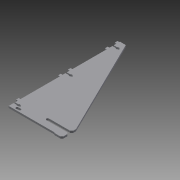
# Autodesk Inventor part: support1
Saved by Autodesk Inventor 2015 SP2 (Build 190223200, 223)
## iProperties
Created: 2016-02-16
Part Number: support1
Material: Generic
Document SubType Name: Modeling
Designer: marc
Density: 1 g/cm^3
Appearance: Default
Author: marc
Autodesk Inventor part; units mm, degrees
ref_plane "YZ Plane" through (0, 0, 0) normal (1, 0, 0) x (0, 1, 0)
ref_plane "XZ Plane" through (0, 0, 0) normal (0, 1, 0) x (-1, 0, 0)
ref_plane "XY Plane" through (0, 0, 0) normal (0, 0, 1) x (1, 0, 0)
sketch "Sketch1" plane through (0, 0, 0) normal (0, 0, 1) x (1, 0, 0)
  line L0 (0, 0) -> (183.9, 0)
  line L1 (183.9, 0) -> (183.9, 47)
  line L2 (183.9, 47) -> (25.4, 370)
  line L3 (25.4, 370) -> (0, 370)
  line L4 (0, 370) -> (0, 0)
  dimension "d0" = 370
  dimension "d1" = 183.9
  dimension "d2" = 25.4
  dimension "d3" = 47
  constraints: 10 end point, 2 perpendicular, 1 horizontal, 1 parallel
  measures "d0" distance between parallel lines of L0 L3
  measures "d1" distance between parallel lines of L1 L4
  measures "d2" distance of L2.end L3.end
  measures "d3" distance of L0.end L1.end
extrude "Extrusion1" add sketch "Sketch1" along normal blind 6
sketch "Sketch2" plane through (0, 0, 6) normal (0, 0, 1) x (1, 0, 0)
  line L0 (0, 370) -> (6, 370)
  line L1 (6, 370) -> (6, 367.743)
  line L2 (6, 367.743) -> (0, 367.743)
  line L3 (0, 367.743) -> (0, 370)
  line L4 (25.4, 370) -> (0, 370) projected
  line L5 (0, 370) -> (0, 0) projected
  line L6 (0, 358.743) -> (6, 358.743)
  line L7 (6, 358.743) -> (6, 335.443)
  line L8 (6, 335.443) -> (0, 335.443)
  line L9 (0, 335.443) -> (0, 358.743)
  line L10 (0, 326.443) -> (6, 326.443)
  line L11 (6, 326.443) -> (6, 212.65)
  line L12 (6, 212.65) -> (0, 212.65)
  line L13 (0, 212.65) -> (0, 326.443)
  line L14 (0, 203.65) -> (6, 203.65)
  line L15 (6, 203.65) -> (6, 180.35)
  line L16 (6, 180.35) -> (0, 180.35)
  line L17 (0, 180.35) -> (0, 203.65)
  line L18 (0, 171.35) -> (6, 171.35)
  line L19 (6, 171.35) -> (6, 41.15)
  line L20 (6, 41.15) -> (0, 41.15)
  line L21 (0, 41.15) -> (0, 171.35)
  line L22 (0, 32.15) -> (6, 32.15)
  line L23 (6, 32.15) -> (6, 0)
  line L24 (6, 0) -> (0, 0)
  line L25 (0, 0) -> (0, 32.15)
  line L26 (0, 0) -> (183.9, 0) projected
  dimension "d6" = 9
  dimension "d7" = 9
  dimension "d8" = 9
  dimension "d9" = 9
  dimension "d12" = 6
  dimension "d14" = 9
  dimension "d53" = 32.15
  dimension "d54" = 171.35
  dimension "d55" = 203.65
  dimension "d56" = 326.443
  dimension "d57" = 358.743
  constraints: 48 end point, 12 parallel, 7 point on line, 6 collinear, 6 horizontal, 6 perpendicular
  measures "d6" distance between parallel lines of L6 L2
  measures "d7" distance between parallel lines of L8 L10
  measures "d8" distance between parallel lines of L22 L20
  measures "d9" distance between parallel lines of L18 L16
  measures "d12" distance between parallel lines of L5 L1
  measures "d14" distance between parallel lines of L12 L14
  measures "d53" distance between parallel lines of L26 L22
  measures "d54" distance between parallel lines of L26 L18
  measures "d55" distance between parallel lines of L26 L14
  measures "d56" distance between parallel lines of L26 L10
  measures "d57" distance between parallel lines of L26 L6
extrude "Extrusion2" cut sketch "Sketch2" against normal through all
sketch "Sketch3" plane through (0, 0, 6) normal (0, 0, 1) x (1, 0, 0)
  line L0 (-10.0727, 347.093) -> (75.5841, 347.093) construction
  line L1 (6, 344.893) -> (27.1, 344.893)
  line L2 (27.1, 344.893) -> (27.1, 349.293)
  line L3 (27.1, 349.293) -> (6, 349.293)
  line L4 (6, 349.293) -> (6, 344.893)
  line L5 (6, 344.893) -> (27.1, 349.293) construction
  line L6 (27.1, 344.893) -> (6, 349.293) construction
  line L7 (6, 358.743) -> (6, 335.443) projected
  line L8 (18, 343.093) -> (23.1, 343.093)
  line L9 (23.1, 343.093) -> (23.1, 351.093)
  line L10 (23.1, 351.093) -> (18, 351.093)
  line L11 (18, 351.093) -> (18, 343.093)
  line L12 (18, 343.093) -> (23.1, 351.093) construction
  line L13 (23.1, 343.093) -> (18, 351.093) construction
  line L14 (25.4, 370) -> (6, 370) projected
  line L15 (-23.1846, 192) -> (187.875, 192) construction
  line L16 (6, 189.8) -> (27.1, 189.8)
  line L17 (27.1, 189.8) -> (27.1, 194.2)
  line L18 (27.1, 194.2) -> (6, 194.2)
  line L19 (6, 194.2) -> (6, 189.8)
  line L20 (6, 189.8) -> (27.1, 194.2) construction
  line L21 (27.1, 189.8) -> (6, 194.2) construction
  line L22 (23.1, 188) -> (18, 188)
  line L23 (18, 188) -> (18, 196)
  line L24 (18, 196) -> (23.1, 196)
  line L25 (23.1, 196) -> (23.1, 188)
  line L26 (23.1, 188) -> (18, 196) construction
  line L27 (18, 188) -> (23.1, 196) construction
  line L28 (6, 203.65) -> (6, 180.35) projected
  line L29 (20.55, 484.1375) -> (20.55, -100.4436) construction
  line L30 (-93.0618, 20.51) -> (253.6101, 20.51) construction
  line L31 (6, 18.31) -> (27.1, 18.31)
  line L32 (27.1, 18.31) -> (27.1, 22.71)
  line L33 (27.1, 22.71) -> (6, 22.71)
  line L34 (6, 22.71) -> (6, 18.31)
  line L35 (6, 18.31) -> (27.1, 22.71) construction
  line L36 (27.1, 18.31) -> (6, 22.71) construction
  line L37 (23.1, 16.51) -> (18, 16.51)
  line L38 (18, 16.51) -> (18, 24.51)
  line L39 (18, 24.51) -> (23.1, 24.51)
  line L40 (23.1, 24.51) -> (23.1, 16.51)
  line L41 (23.1, 16.51) -> (18, 24.51) construction
  line L42 (18, 16.51) -> (23.1, 24.51) construction
  line L43 (6, 32.15) -> (6, 0) projected
  line L44 (6, 0) -> (183.9, 0) projected
  point P0 (0, 0)
  point P1 (16.55, 347.093)
  point P2 (20.55, 347.093)
  point P3 (16.55, 192)
  point P4 (20.55, 192)
  point P5 (20.55, 347.093)
  point P6 (20.55, 192)
  point P7 (16.55, 20.51)
  point P8 (20.55, 20.51)
  point P9 (20.55, 20.51)
  dimension "d20" = 5.1
  dimension "d21" = 4.4
  dimension "d22" = 17.1
  dimension "d23" = 21.1
  dimension "d25" = 8
  dimension "d58" = 192
  dimension "d59" = 20.51
  dimension "d60" = 347.093
  constraints: 80 end point, 15 midpoint, 12 parallel, 9 horizontal, 9 point on line, 8 equal length, 6 perpendicular, 3 collinear, 1 vertical
  measures "d20" distance of L8.start L8.end
  measures "d21" distance between parallel lines of L1 L3
  measures "d22" distance between parallel lines of L7 L9
  measures "d23" distance of L2.end L3.end
  measures "d25" distance between parallel lines of L8 L10
  measures "d58" distance between parallel lines of L44 L15
  measures "d59" distance between parallel lines of L44 L30
  measures "d60" distance between parallel lines of L44 L0
extrude "Extrusion3" cut sketch "Sketch3" against normal through all
sketch "Sketch4" plane through (0, 0, 6) normal (0, 0, 1) x (1, 0, 0)
  line L0 (6, 0) -> (156.8, 0)
  line L1 (156.8, 0) -> (156.8, 2)
  line L2 (156.8, 2) -> (6, 2)
  line L3 (6, 2) -> (6, 0)
  point P0 (0, 0)
  dimension "d35" = 2
  dimension "d36" = 150.8
  constraints: 8 end point, 2 parallel, 1 horizontal, 1 perpendicular
  measures "d35" distance between parallel lines of L0 L2
  measures "d36" distance from line of L0.start L1
extrude "Extrusion4" cut sketch "Sketch4" against normal through all
sketch "Sketch5" plane through (0, 0, 6) normal (0, 0, 1) x (1, 0, 0)
  line L0 (70.0249, 28) -> (233.8249, 28) construction
  line L1 (108.9, 23.6) -> (183.9, 23.6)
  line L2 (183.9, 23.6) -> (183.9, 32.4)
  line L3 (183.9, 32.4) -> (108.9, 32.4)
  line L4 (108.9, 32.4) -> (108.9, 23.6)
  line L5 (108.9, 23.6) -> (183.9, 32.4) construction
  line L6 (183.9, 23.6) -> (108.9, 32.4) construction
  line L7 (183.9, 0) -> (183.9, 47) projected
  line L8 (156.8, 0) -> (183.9, 0) projected
  circle A0 centre (108.9, 28) radius 4.37
  point P0 (0, 0)
  point P1 (146.4, 28)
  point P2 (183.9, 2)
  dimension "d34" = 8.8
  dimension "d37" = 28
  dimension "d38" = 75
  constraints: 14 end point, 3 midpoint, 2 horizontal, 2 parallel, 1 centre point, 1 collinear, 1 perpendicular, 1 point on line, 1 tangent
  measures "d34" distance between parallel lines of L1 L3
  measures "d37" distance between parallel lines of L8 L0
  measures "d38" distance of L2.end L3.end
extrude "Extrusion5" cut sketch "Sketch5" against normal through all
sketch "Sketch6" plane through (0, 0, 6) normal (0, 0, 1) x (1, 0, 0)
  line L0 (26, 6) -> (34, 6)
  line L1 (34, 6) -> (34, 14)
  line L2 (34, 14) -> (26, 14)
  line L3 (26, 14) -> (26, 6)
  line L4 (26, 6) -> (34, 14) construction
  line L5 (34, 6) -> (26, 14) construction
  circle A0 centre (26, 10) radius 4
  circle A1 centre (34, 10) radius 4
  line L6 (6, 2) -> (156.8, 2) projected
  line L7 (6, 18.31) -> (6, 2) projected
  point P0 (0, 0)
  point P1 (30, 10)
  dimension "d41" = 8
  dimension "d42" = 8
  dimension "d43" = 8
  dimension "d44" = 24
  constraints: 12 end point, 4 midpoint, 2 centre point, 2 parallel, 2 tangent, 1 horizontal, 1 perpendicular
  measures "d41" distance from line of L6 point (30, 10)
  measures "d42" distance of L1.end L2.end
  measures "d43" distance between parallel lines of L0 L2
  measures "d44" distance from line of L7 point (30, 10)
extrude "Extrusion6" cut sketch "Sketch6" against normal through all
chamfer "Chamfer1" distance 2 angle 45 1 edges at (156.8, 0, 3)
chamfer "Chamfer2" distance 5 angle 45 3 edges at (183.9, 32.4, 3) (183.9, 23.6, 3) (183.9, 0, 3)
body "Solid1"
